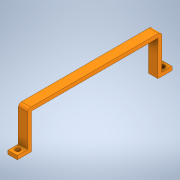
# Autodesk Inventor part: battery_pack_clamp
Saved by Autodesk Inventor 2020.3 (Build 243373000, 373)
## iProperties
Created: 2020-07-02
Part Number: battery_pack_clamp
Material: PET Plastic
Document SubType Name: Modeling
Designer: Devin
Density: 1.541 g/cm^3
Appearance: Orange
Author: Devin
Autodesk Inventor part; units mm, degrees
ref_plane "YZ Plane" through (0, 0, 0) normal (1, 0, 0) x (0, 1, 0)
ref_plane "XZ Plane" through (0, 0, 0) normal (0, 1, 0) x (-1, 0, 0)
ref_plane "XY Plane" through (0, 0, 0) normal (0, 0, 1) x (1, 0, 0)
sketch "Sketch1" plane through (0, 0, 0) normal (1, 0, 0) x (0, 1, 0)
  line L0 (0, 0) -> (0, -80.85)
  line L1 (0, 0) -> (-22.5, 0)
  line L2 (-22.5, 0) -> (-22.5, 9)
  line L3 (-22.5, 9) -> (-20.1, 9)
  line L4 (-20.1, 9) -> (-20.1, 2.4)
  line L5 (-20.1, 2.4) -> (2.4, 2.4)
  line L6 (2.4, 2.4) -> (2.4, -40.425)
  line L7 (0, -80.85) -> (-22.5, -80.85)
  line L8 (-22.5, -80.85) -> (-22.5, -89.85)
  line L9 (-22.5, -89.85) -> (-20.1, -89.85)
  line L10 (-20.1, -89.85) -> (-20.1, -83.25)
  line L11 (-20.1, -83.25) -> (2.4, -83.25)
  line L12 (2.4, -83.25) -> (2.4, -40.425)
  dimension "d0" = 80.85
  dimension "d17" = 22.5
  dimension "d18" = 9
  dimension "d19" = 2.4
  dimension "d20" = 6.6
  dimension "d21" = 22.5
  dimension "d23" = 2.4
  dimension "d24" = 2.4
  dimension "d25" = 9
  dimension "d26" = 2.4
  constraints: 26 end point, 4 perpendicular, 1 horizontal, 1 vertical
  measures "d0" distance of L0.start L0.end
  measures "d17" distance of L0.start L1.end
  measures "d18" distance of L1.end L2.end
  measures "d19" distance of L2.end L3.end
  measures "d20" distance of L3.end L4.end
  measures "d21" distance of L4.end L5.end
  measures "d23" distance between parallel lines of L7 L11
  measures "d24" distance between parallel lines of L0 L12
  measures "d25" distance between parallel lines of L9 L7
  measures "d26" distance between parallel lines of L10 L8
extrude "Extrusion1" add sketch "Sketch1" along normal blind 6
fillet "Fillet1" radius 2 1 edges at (3, 2.4, 2.4)
fillet "Fillet2" radius 2 1 edges at (3, 2.4, -83.25)
sketch "Sketch3" plane through (0, -20.1, 9) normal (0, 1, 0) x (1, 0, 0)
  line L0 (0, 6.6) -> (0, 0) projected
  line L1 (0, 6.6) -> (6, 6.6) projected
  circle A0 centre (3, 3.3) radius 1.55
  line L2 (0, 92.25) -> (6, 92.25) projected
  line L3 (6, 98.85) -> (6, 92.25) projected
  circle A1 centre (3, 95.55) radius 1.55
  line L4 (0, 0) -> (6, 0) projected
  line L5 (0, 98.85) -> (0, 92.25) projected
  point P0 (0, 9)
  dimension "d29" = 3.1
  dimension "d30" = 3.1
  constraints: 2 centre point
  measures "d29" diameter of A0
  measures "d30" diameter of A1
extrude "Extrusion3" cut sketch "Sketch3" against normal blind 10
body "Solid1"
